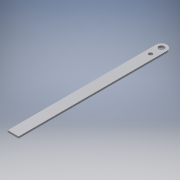
# Autodesk Inventor part: columna01
Saved by Autodesk Inventor 2016 (Build 200138000, 138)
## iProperties
Created: 2016-09-08
Part Number: columna01
Material: Madera (abedul)
Document SubType Name: Modeling
Designer: Iván
Density: 0.55 g/cm^3
Appearance: Suave - Blanco
Author: Iván
Autodesk Inventor part; units mm, degrees
ref_plane "YZ Plane" through (0, 0, 0) normal (1, 0, 0) x (0, 1, 0)
ref_plane "XZ Plane" through (0, 0, 0) normal (0, 1, 0) x (-1, 0, 0)
ref_plane "XY Plane" through (0, 0, 0) normal (0, 0, 1) x (1, 0, 0)
sketch "Boceto1" plane through (0, 0, 0) normal (0, 0, 1) x (1, 0, 0)
  line L0 (0, 0) -> (25, 0)
  line L1 (12.5, 0) -> (12.5, 340)
  circle A0 centre (12.5, 340) radius 6.5
  circle A1 centre (12.5, 340) radius 12.5
  line L2 (25, 340) -> (25, 0)
  line L3 (0, 0) -> (0, 340)
  line L4 (12.5, 340) -> (12.5, 315.2)
  circle A2 centre (12.5, 315.2) radius 4.4
  dimension "d0" = 25
  dimension "d8" = 340
  dimension "d9" = 13
  dimension "d10" = 25
  dimension "d13" = 24.8
  dimension "d14" = 8.8
  constraints: 10 end point, 3 centre point, 3 coincident, 2 point on circle, 2 tangent, 1 horizontal, 1 midpoint, 1 point on line, 1 vertical
  measures "d0" distance of L0.start L0.end
  measures "d8" distance of L1.start L1.end
  measures "d9" diameter of A0
  measures "d10" diameter of A1
  measures "d13" distance of L4.start L4.end
  measures "d14" diameter of A2
extrude "Extrusión2" add sketch "Boceto1" along normal blind 4 contours L3 A1 L1 A2 L0 | L1 A2 A1 L2 L0 | A1
